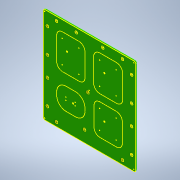
# Autodesk Inventor part: OCU_PCB
Saved by Autodesk Inventor 2021 (Build 250183000, 183)
## iProperties
Created: 2020-11-06
Part Number: OCU_PCB
Material: Generic
Document SubType Name: Modeling
Designer: lgnds
Density: 1 g/cm^3
Appearance: Default
Author: lgnds
Autodesk Inventor part; units mm, degrees
ref_plane "YZ Plane" through (0, 0, 0) normal (1, 0, 0) x (0, 1, 0)
ref_plane "XZ Plane" through (0, 0, 0) normal (0, 1, 0) x (-1, 0, 0)
ref_plane "XY Plane" through (0, 0, 0) normal (0, 0, 1) x (1, 0, 0)
sketch "Sketch1" plane through (0, 0, 0) normal (0, 0, 1) x (1, 0, 0)
  line L0 (-56, -58) -> (56, -58)
  line L1 (56, -58) -> (56, 58)
  line L2 (56, 58) -> (-56, 58)
  line L3 (-56, 58) -> (-56, -58)
  line L4 (-56, -58) -> (56, 58) construction
  line L5 (56, -58) -> (-56, 58) construction
  point P0 (0, 0)
  dimension "d0" = 116
  dimension "d1" = 112
  constraints: 12 end point, 2 midpoint, 2 parallel, 1 horizontal, 1 perpendicular
  measures "d0" distance between parallel lines of L0 L2
  measures "d1" distance between parallel lines of L1 L3
extrude "Extrusion1" add sketch "Sketch1" along normal blind 1.6
fillet "Fillet1" radius 2 4 edges at (-56, 58, 0.8) (-56, -58, 0.8) (56, -58, 0.8) (56, 58, 0.8)
sketch "Sketch5" plane through (0, 0, 1.6) normal (0, 0, 1) x (1, 0, 0)
  circle A0 centre (-2, -3) radius 1.6
  circle A1 centre (-6, -44) radius 1.6
  circle A2 centre (40, -53) radius 1.6
  circle A3 centre (51, -42) radius 1.6
  circle A4 centre (51, -12) radius 1.6
  line L0 (56, -56) -> (56, 56) construction
  line L1 (-54, -58) -> (54, -58) construction
  line L2 (0, 81.2) -> (0, -81.2) construction
  line L3 (-78.4, 0) -> (78.4, 0) construction
  circle A5 centre (-40, -53) radius 1.6
  circle A6 centre (-51, -42) radius 1.6
  circle A7 centre (-51, -12) radius 1.6
  circle A8 centre (40, 53) radius 1.6
  circle A9 centre (51, 42) radius 1.6
  circle A10 centre (51, 12) radius 1.6
  line L4 (-54, 58) -> (54, 58) construction
  circle A11 centre (-51, 12) radius 1.6
  circle A12 centre (-51, 42) radius 1.6
  circle A13 centre (-40, 53) radius 1.6
  circle A14 centre (16, 53) radius 1.6
  circle A15 centre (-16, 53) radius 1.6
  point P0 (0, 0)
  point P1 (-56, -56)
  point P2 (-56, 56)
  dimension "d19" = 44
  dimension "d20" = 6
  dimension "d21" = 3
  dimension "d22" = 2
  dimension "d23" = 5
  dimension "d24" = 5
  dimension "d25" = 5
  dimension "d27" = 3.2
  dimension "d28" = 3.2
  dimension "d29" = 3.2
  dimension "d31" = 3.2
  dimension "d32" = 3.2
  dimension "d33" = 16
  dimension "d34" = 16
  dimension "d35" = 12
  dimension "d36" = 3.2
  dimension "d37" = 3.2
  dimension "d38" = 5
  dimension "d39" = 5
  dimension "d40" = 16
  dimension "d41" = 16
  constraints: 16 centre point, 13 symmetric about line, 2 end point, 9 other
  measures "d19" vertical distance of point (0, 0) A1.centre
  measures "d20" horizontal distance of point (0, 0) A1.centre
  measures "d21" vertical distance of point (0, 0) A0.centre
  measures "d22" horizontal distance of point (0, 0) A0.centre
  measures "d23" distance from line of L0 A4.centre
  measures "d24" distance from line of L0 A3.centre
  measures "d25" distance from line of L1 A2.centre
  measures "d27" diameter of A4
  measures "d28" diameter of A3
  measures "d29" diameter of A2
  measures "d31" diameter of A0
  measures "d32" diameter of A1
  measures "d33" distance from line of L0 A2.centre
  measures "d34" distance from line of L1 A3.centre
  measures "d35" vertical distance of point (0, 0) A4.centre
  measures "d36" diameter of A15
  measures "d37" diameter of A14
  measures "d38" distance from line of L4 A14.centre
  measures "d39" distance from line of L4 A15.centre
  measures "d40" distance from line of L2 A14.centre
  measures "d41" distance from line of L2 A15.centre
extrude "Extrusion4" cut sketch "Sketch5" against normal through all
sketch "OCU_PCB_OUTLINE" plane through (0, 0, 1.6) normal (0, 0, 1) x (1, 0, 0)
  circle A0 centre (18.0683, -23.4912) radius 0.7836 projected
  circle A1 centre (-27.1869, 27.3078) radius 0.7836 projected
  circle A2 centre (18.0683, 27.3078) radius 0.7836 projected
  line L0 (32.6352, -42.846) -> (12.62, -42.846) projected
  line L1 (32.6352, -42.846) -> (12.62, -42.846) projected
  arc A3 (32.6352, -42.846) -> (39.7472, -35.734) centre (32.6352, -35.734) ccw projected
  line L2 (39.7472, -12.62) -> (39.7472, -35.734) projected
  arc A4 (39.7472, -12.62) -> (32.6352, -5.508) centre (32.6352, -12.62) ccw projected
  line L3 (12.62, -5.508) -> (32.6352, -5.508) projected
  arc A5 (12.62, -5.508) -> (5.508, -12.62) centre (12.62, -12.62) ccw projected
  line L4 (5.508, -35.734) -> (5.508, -12.62) projected
  arc A6 (5.508, -35.734) -> (12.62, -42.846) centre (12.62, -35.734) ccw projected
  arc A7 (-16.9126, -36.0388) -> (-5.4826, -24.6088) centre (-16.9126, -24.6088) ccw projected
  arc A8 (-16.9126, -36.0388) -> (-5.4826, -24.6088) centre (-16.9126, -24.6088) ccw projected
  line L5 (-5.4826, -21.0528) -> (-5.4826, -24.6088) projected
  arc A9 (-5.4826, -21.0528) -> (-16.9126, -9.6228) centre (-16.9126, -21.0528) ccw projected
  line L6 (-28.3426, -9.6228) -> (-16.9126, -9.6228) projected
  arc A10 (-28.3426, -9.6228) -> (-39.7726, -21.0528) centre (-28.3426, -21.0528) ccw projected
  line L7 (-39.7726, -24.6088) -> (-39.7726, -21.0528) projected
  arc A11 (-39.7726, -24.6088) -> (-28.3426, -36.0388) centre (-28.3426, -24.6088) ccw projected
  line L8 (-16.9126, -36.0388) -> (-28.3426, -36.0388) projected
  arc A12 (-12.62, 3.508) -> (-5.508, 10.62) centre (-12.62, 10.62) ccw projected
  arc A13 (-12.62, 3.508) -> (-5.508, 10.62) centre (-12.62, 10.62) ccw projected
  line L9 (-5.508, 38.179) -> (-5.508, 10.62) projected
  arc A14 (-5.508, 38.179) -> (-12.62, 45.291) centre (-12.62, 38.179) ccw projected
  line L10 (-32.6352, 45.291) -> (-12.62, 45.291) projected
  arc A15 (-32.6352, 45.291) -> (-39.7472, 38.179) centre (-32.6352, 38.179) ccw projected
  line L11 (-39.7472, 10.62) -> (-39.7472, 38.179) projected
  arc A16 (-39.7472, 10.62) -> (-32.6352, 3.508) centre (-32.6352, 10.62) ccw projected
  line L12 (-12.62, 3.508) -> (-32.6352, 3.508) projected
  arc A17 (5, 10.62) -> (12.62, 3) centre (12.62, 10.62) ccw projected
  arc A18 (5, 10.62) -> (12.62, 3) centre (12.62, 10.62) ccw projected
  line L13 (32.6352, 3) -> (12.62, 3) projected
  arc A19 (32.6352, 3) -> (40.2552, 10.62) centre (32.6352, 10.62) ccw projected
  line L14 (40.2552, 38.179) -> (40.2552, 10.62) projected
  arc A20 (40.2552, 38.179) -> (32.6352, 45.799) centre (32.6352, 38.179) ccw projected
  line L15 (12.62, 45.799) -> (32.6352, 45.799) projected
  arc A21 (12.62, 45.799) -> (5, 38.179) centre (12.62, 38.179) ccw projected
  line L16 (5, 10.62) -> (5, 38.179) projected
  circle A22 centre (-19.8971, -23.4785) radius 0.7836 projected
  circle A23 centre (51, -42) radius 1.6 projected
  circle A24 centre (-51, -42) radius 1.6 projected
  circle A25 centre (-51, 42) radius 1.6 projected
  circle A26 centre (51, 42) radius 1.6 projected
  circle A27 centre (40, 53) radius 1.6 projected
  circle A28 centre (-51, 12) radius 1.6 projected
  circle A29 centre (-40, -53) radius 1.6 projected
  circle A30 centre (40, -53) radius 1.6 projected
  circle A31 centre (51, -12) radius 1.6 projected
  circle A32 centre (-51, -12) radius 1.6 projected
  circle A33 centre (-40, 53) radius 1.6 projected
  circle A34 centre (51, 12) radius 1.6 projected
  circle A35 centre (16, 53) radius 1.6 projected
  circle A36 centre (-2, -3) radius 1.6 projected
  circle A37 centre (-6, -44) radius 1.6 projected
  circle A38 centre (-16, 53) radius 1.6 projected
  arc A39 (56, 56) -> (54, 58) centre (54, 56) ccw projected
  line L17 (54, 58) -> (-54, 58) projected
  arc A40 (-54, 58) -> (-56, 56) centre (-54, 56) ccw projected
  line L18 (-56, 56) -> (-56, -56) projected
  arc A41 (-56, -56) -> (-54, -58) centre (-54, -56) ccw projected
  line L19 (-54, -58) -> (54, -58) projected
  arc A42 (54, -58) -> (56, -56) centre (54, -56) ccw projected
  line L20 (56, -56) -> (56, 56) projected
  point P0 (0, 0)
equation "\"d24\" = d23"
equation "\"d25\" = d23"
equation "\"d28\" = d27"
equation "\"d29\" = d27"
equation "\"d31\" = d27"
equation "\"d32\" = d27"
equation "\"d36\" = d27"
equation "\"d37\" = d27"
equation "\"d38\" = d23"
equation "\"d39\" = d23"
equation "\"d40\" = d34"
equation "\"d41\" = d34"
body "Solid1"
